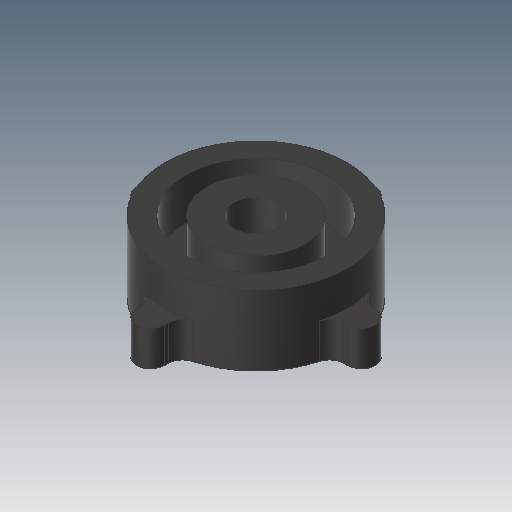
# Autodesk Inventor part: lod_base
Saved by Autodesk Inventor 2019.4 (Build 234330000, 330)
## iProperties
Created: 2018-07-25
Part Number: lod_base
Material: ABS プラスチック
Document SubType Name: Modeling
Designer: y6tada
Density: 1.06 g/cm^3
Appearance: 滑らか - 黒
Mass: 0.574452 g
Surface Area: 7.22766 cm^2
Volume: 0.541936 cm^3
Author: y6tada
Autodesk Inventor part; units mm, degrees
ref_plane "YZ Plane" through (0, 0, 0) normal (1, 0, 0) x (0, 1, 0)
ref_plane "XZ Plane" through (0, 0, 0) normal (0, 1, 0) x (-1, 0, 0)
ref_plane "XY Plane" through (0, 0, 0) normal (0, 0, 1) x (1, 0, 0)
sketch "スケッチ1" plane through (0, 0, 0) normal (0, 1, 0) x (-1, 0, 0)
  arc A0 (6.2646, 1.7333) -> (1.7333, 6.2646) centre (0, 0) ccw
  arc A1 (1, 7.5) -> (0, 8.5) centre (0, 7.5) ccw
  line L0 (1, 7.5) -> (1, 7.2284)
  line L1 (0, 1.6) -> (0, 7.5)
  line L2 (0, 7.5) -> (0, 8.5)
  line L3 (1.6, 0) -> (7.5, 0)
  line L4 (7.5, 0) -> (8.5, 0)
  arc A2 (8.5, 0) -> (7.5, 1) centre (7.5, 0) ccw
  line L5 (7.5, 1) -> (7.2284, 1)
  arc A3 (7.5, 0) -> (0, 7.5) centre (0, 0) ccw construction
  arc A4 (1, 7.2284) -> (1.7333, 6.2646) centre (2, 7.2284) ccw
  arc A5 (6.2646, 1.7333) -> (7.2284, 1) centre (7.2284, 2) ccw
  arc A6 (1.6, 0) -> (0, 1.6) centre (0, 0) ccw
  point P0 (6.4226, 1)
  point P1 (1, 6.4226)
  dimension "d0" = 1
  dimension "d1" = 6.5
  dimension "d2" = 1
  dimension "d4" = 7.5
  dimension "d18" = 1.6
  constraints: 16 point on circle, 12 end point, 7 centre point, 6 tangent, 5 point on line, 4 coincident, 2 equal radius, 2 horizontal, 2 vertical, 1 collinear
  measures "d0" radius of A2
  measures "d1" radius of A0
  measures "d2" radius of A4
  measures "d4" radius of A3
  measures "d18" radius of A6
extrude "押し出し1" add sketch "スケッチ1" along normal blind 5
pattern_circular "円形状パターン1" count 4 over 360 about axis through (0, -10, 0) along (0, 1, 0) of "押し出し1"
sketch "スケッチ2" plane through (0, 5, 0) normal (0, 1, 0) x (1, 0, 0)
  circle A0 centre (0, 0) radius 5
  circle A1 centre (0, 0) radius 3.5
  dimension "d10" = 1.5
  dimension "d11" = 10
  constraints: 2 centre point, 2 coincident
  measures "d10" radial gap between concentric circles of A1 A0
  measures "d11" diameter of A0
extrude "押し出し3" cut sketch "スケッチ2" against normal blind 3
sketch "スケッチ3" plane through (0, 5, 0) normal (0, 1, 0) x (1, 0, 0)
  circle A0 centre (0, 0) radius 8.5
  arc A1 (-6.2646, -1.7333) -> (-1.7333, -6.2646) centre (0, 0) ccw construction
  circle A2 centre (0, 0) radius 6.5
  arc A3 (-1, -7.5) -> (1, -7.5) centre (0, -7.5) ccw construction
  constraints: 2 coincident, 1 centre point, 1 tangent, 3 other
extrude "押し出し4" cut sketch "スケッチ3" against normal blind 2.5
